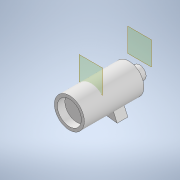
# Autodesk Inventor part: ReverserClicker
Saved by Autodesk Inventor 2021 (Build 250183000, 183)
## iProperties
Created: 2021-07-19
Part Number: ReverserClicker
Material: Generic
Document SubType Name: Modeling
Designer: teh18
Density: 1 g/cm^3
Appearance: Default
Author: teh18
Autodesk Inventor part; units mm, degrees
ref_plane "YZ Plane" through (0, 0, 0) normal (1, 0, 0) x (0, 1, 0)
ref_plane "XZ Plane" through (0, 0, 0) normal (0, 1, 0) x (-1, 0, 0)
ref_plane "XY Plane" through (0, 0, 0) normal (0, 0, 1) x (1, 0, 0)
ref_plane "Work Plane3" through (-4, -4, -10) normal (0, 0, -1) x (0, 1, 0)
ref_plane "Work Plane6" through (0, 0, -10) normal (0, 0, -1) x (-1, 0, 0)
ref_plane "Work Plane4" through (-20.0043, -85.0498, -55.625) normal (0, 0, -1) x (0, 1, 0)
ref_plane "Work Plane5" through (0, 0, -55.625) normal (0, 0, -1) x (-1, 0, 0)
sketch "Sketch6" plane through (0, 0, -55.625) normal (0, 0, -1) x (-1, 0, 0)
  arc A0 (75.4786, 4.8454) -> (74.2911, 5.1636) centre (74.7523, 4.5099) ccw projected
  arc A1 (56.7048, 9.4732) -> (74.2911, 5.1636) centre (67.3726, 14.9684) ccw projected
  line L0 (55.5232, 13.0737) -> (56.7048, 9.4732) projected
  arc A2 (55.5232, 13.0737) -> (41.5887, -50.9456) centre (67.3725, -23.0316) ccw projected
  line L1 (33.4464, -59.7606) -> (41.5887, -50.9456) projected
  arc A3 (33.4464, -59.7606) -> (104.1015, -56.9577) centre (67.3725, -23.0316) ccw projected
  line L2 (112.9165, -65.0999) -> (104.1015, -56.9577) projected
  arc A4 (112.9165, -65.0999) -> (124.3718, -47.4258) centre (67.3725, -23.0316) ccw projected
  line L3 (113.3397, -42.7043) -> (124.3718, -47.4258) projected
  arc A5 (113.3397, -42.7043) -> (116.0567, -34.4268) centre (67.3725, -23.0316) ccw projected
  arc A6 (116.0567, -34.4268) -> (112.8612, -32.4083) centre (114.1093, -33.971) ccw projected
  arc A7 (103.4777, -34.8812) -> (112.8612, -32.4083) centre (105.3725, -23.0317) ccw projected
  line L4 (99.8772, -33.6995) -> (103.4777, -34.8812) projected
  arc A8 (95.5677, -16.1132) -> (99.8772, -33.6995) centre (105.3725, -23.0317) ccw projected
  arc A9 (95.5677, -16.1132) -> (95.2495, -14.9257) centre (94.9141, -15.652) ccw projected
  arc A10 (88.3311, -2.9425) -> (95.2495, -14.9257) centre (100.2815, -4.0317) ccw projected
  arc A11 (88.3311, -2.9425) -> (87.4618, -2.0732) centre (87.5344, -2.8699) ccw projected
  arc A12 (75.4786, 4.8454) -> (87.4618, -2.0732) centre (86.3726, 9.8773) ccw projected
  circle A13 centre (67.3725, -23.0316) radius 18 projected
  circle A14 centre (0, 0) radius 2.7453
  line L5 (41.5887, -50.9456) -> (4.0711, -16.2912)
  line L6 (33.4464, -59.7606) -> (-4.0711, -25.1062)
  line L7 (-32.6275, -120.0316) -> (-32.6275, 19.9684) projected
  line L8 (-32.6275, 19.9684) -> (137.3725, 19.9684) projected
  line L9 (-1.1617, -56.4813) -> (14.3417, -55.1521) projected
  line L10 (10.9499, -62.3928) -> (18.9164, -61.7098) projected
  line L11 (12.3158, -75.8007) -> (18.9164, -61.7098) projected
  line L12 (14.3417, -55.1521) -> (10.9499, -62.3928) projected
  line L13 (10.9499, -62.3928) -> (33.4464, -59.7606)
  line L14 (10.9499, -62.3928) -> (18.6047, -46.0515)
  line L15 (33.4464, -59.7606) -> (41.5887, -50.9456)
  circle A15 centre (0, -20.6987) radius 6
  constraints: 10 end point, 3 tangent, 2 centre point, 2 collinear, 2 point on circle, 1 coincident, 1 parallel, 1 point on line, 1 vertical alignment
extrude "Extrusion5" add sketch "Sketch6" against normal blind 10 contours L1 L6 A15 L5 | L13 L12 L14 L6 | A15
sketch "Sketch7" plane through (0, -20.6987, -45.625) normal (0, 0, 1) x (1, 0, 0)
  circle A0 centre (0, 0) radius 11.2
  circle A1 centre (0, 0) radius 14
  point P0 (0, 20.6987)
  dimension "d14" = 22.4
  dimension "d15" = 28
  constraints: 2 centre point, 1 coincident
  measures "d14" diameter of A0
  measures "d15" diameter of A1
ref_plane "Work Plane7" through (-4, -24.6987, -7) normal (0, 0, -1) x (0, 1, 0)
extrude "Extrusion6" add sketch "Sketch7" along normal blind 48.625 contours A0 | A1
sketch "Sketch8" plane through (0, -20.6987, 3) normal (0, 0, 1) x (1, 0, 0)
  circle A0 centre (0, 0) radius 4
  circle A1 centre (0, 0) radius 11.2
  circle A2 centre (0, 0) radius 14 projected
  point P0 (0, 20.6987)
  dimension "d18" = 8
  dimension "d19" = 22.4
  constraints: 2 centre point, 1 coincident
  measures "d18" diameter of A0
  measures "d19" diameter of A1
extrude "Extrusion7" add sketch "Sketch8" along normal blind 7 contours A2
ref_plane "Work Plane8" through (-11.409, -39.4049, -55.625) normal (-0.7345804, -0.6785217, 0) x (0, 0, 1)
sketch "Sketch10" plane through (-11.409, -39.4049, -55.625) normal (-0.7345804, -0.6785217, 0) x (0, 0, 1)
  line L0 (0, 0) -> (0, 12) projected
  line L1 (0, 12) -> (10, 12)
  line L2 (10, 12) -> (10, 0)
  line L3 (10, 0) -> (0, 0)
  line L4 (0, 0) -> (0, 12)
  line L5 (2, 0) -> (2, -8)
  line L6 (2, -8) -> (7, -8)
  line L7 (7, -8) -> (7, -4)
  line L8 (7, -4) -> (5, -6)
  line L9 (5, -6) -> (4, -6)
  line L10 (4, -6) -> (4, 0)
  line L11 (6, 0) -> (6, -8)
  line L12 (6, -8) -> (1, -8)
  line L13 (1, -8) -> (1, -4)
  line L14 (1, -4) -> (3, -6)
  line L15 (3, -6) -> (4, -6)
  point P0 (55.625, 21.2048)
  point P1 (6, 0)
  point P2 (2, -5)
  point P3 (6, -8)
  dimension "d23" = 8
  dimension "d24" = 5
  dimension "d25" = 4
  dimension "d26" = 45
  dimension "d27" = 2
  dimension "d28" = 2
  dimension "d29" = 2
  constraints: 30 end point, 5 symmetric about line, 4 perpendicular, 3 parallel, 2 point on line, 1 horizontal, 1 vertical
  measures "d23" distance of L5.start L5.end
  measures "d24" distance of L5.end L6.end
  measures "d25" distance of L6.end L7.end
  measures "d26" angle of L7 L8
  measures "d27" distance between parallel lines of L5 L0
  measures "d28" distance between parallel lines of L6 L9
  measures "d29" distance between parallel lines of L5 L10
extrude "Extrusion8" add sketch "Sketch10" along normal mid plane 8 contours L3 L11 L8 L9 L10 | L14 L15 L9 L8 L11 L6 L5
body "Solid2"
